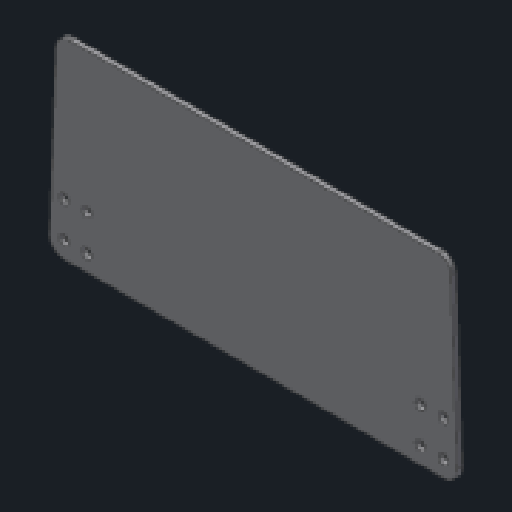
# Autodesk Inventor part: ChestMiddle
Saved by Autodesk Inventor 2025.2 (Build 292293000, 293)
## iProperties
Created: 2025-02-27
Part Number: ChestMiddle
Material: Generic
Document SubType Name: Sheet Metal
Designer: valer
Density: 1 g/cm^3
Sheet Metal Rule: Default
Appearance: Default
Author: valer
Autodesk Inventor part; units mm, degrees
ref_plane "YZ Plane" through (0, 0, 0) normal (1, 0, 0) x (0, 1, 0)
ref_plane "XZ Plane" through (0, 0, 0) normal (0, 1, 0) x (-1, 0, 0)
ref_plane "XY Plane" through (0, 0, 0) normal (0, 0, 1) x (1, 0, 0)
sketch "Sketch1" plane through (0, 0, 0) normal (0, 0, 1) x (1, 0, 0)
  line L0 (248.4589, 0) -> (238.1573, 295) construction
  line L1 (0, 0) -> (10.3016, 295) construction
  line L2 (10.3016, 295) -> (238.1573, 295) construction
  line L3 (248.4589, 0) -> (0, 0) construction
  line L4 (4.2145, 279) -> (244.2444, 279)
  line L5 (244.2444, 279) -> (248.3301, 162)
  line L6 (248.3301, 162) -> (0.1288, 162)
  line L7 (0.1288, 162) -> (4.2145, 279)
  dimension "d0" = 16
  dimension "d5" = 5.525
  dimension "d6" = 5.525
  dimension "d7" = 162
  measures "d0" distance between parallel lines of L2 L4
  measures "d5" distance between parallel lines of L5 L0
  measures "d6" distance between parallel lines of L1 L7
  measures "d7" distance from line of L6 L0.start
extrude "Plate1" add sketch "Sketch1" along normal blind 3.048
fillet "Fillet1" radius 8 4 edges at (248.3301, 162, 1.524) (244.2444, 279, 1.524) (0.1288, 162, 1.524) (4.2145, 279, 1.524)
sketch "Sketch3" plane through (0, 0, 0) normal (0, 0, -1) x (-1, 0, 0)
  circle A0 centre (-225.6616, 172) radius 3 projected
  circle A1 centre (-239.5656, 172) radius 3 projected
  circle A2 centre (-239.5656, 193.718) radius 3 projected
  circle A3 centre (-225.6616, 193.718) radius 3 projected
  line L0 (-240.0459, 162) -> (-8.413, 162) projected
  line L1 (-124.2295, 162) -> (-124.2295, 279)
  line L2 (-11.94, 279) -> (-236.5189, 279) projected
  circle A4 centre (-22.7973, 172) radius 3
  circle A5 centre (-8.8933, 172) radius 3
  circle A6 centre (-8.8933, 193.718) radius 3
  circle A7 centre (-22.7973, 193.718) radius 3
  point P0 (0, 0)
  constraints: 4 centre point, 4 symmetric about line, 2 end point, 2 midpoint, 4 other
extrude "Cut2" cut sketch "Sketch3" against normal blind 3.048
equation "\"d6\" = d5"
equation "\"d25\" = Thickness"
equation "\"d4\" = Thickness"
equation "\"BendRadius\" = Thickness"
equation "\"BendReliefWidth\" = Thickness"
equation "\"BendReliefDepth\" = 0.5 * Thickness"
equation "\"CornerReliefSize\" = 4 * Thickness"
equation "\"MinimumRemnant\" = 2 * Thickness"
equation "\"TransitionRadius\" = BendRadius"
equation "\"JacobiRadiusSize\" = BendRadius"
equation "\"GapSize\" = Thickness"
equation "\"Thickness\" = 3.048"
body "Solid1"
